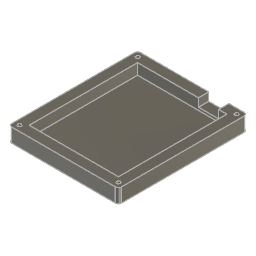
hackpad (Autodesk Fusion 360 archive; units mm, degrees)
design "case_bottom"
part number: 2026-02-01-13-29-20-341
part number: 2026-02-01-13-33-14-051
Autodesk Fusion 360 part; units mm, degrees
sketch "Sketch1" plane through (0, 0, 0) normal (0, 0, 1) x (1, 0, 0) in component "Oliver's Epic Mathpad"
  line L0 (-38.0199, 45) -> (43.9801, 45)
  line L1 (43.9801, 45) -> (43.9801, -54.6)
  line L2 (43.9801, -54.6) -> (-38.0199, -54.6)
  line L3 (-38.0199, -54.6) -> (-38.0199, 45)
  line L4 (-47.5199, 54.5) -> (53.4801, 54.5)
  line L5 (53.4801, 54.5) -> (53.4801, -64.1)
  line L6 (53.4801, -64.1) -> (-47.5199, -64.1)
  line L7 (-47.5199, -64.1) -> (-47.5199, 54.5)
  circle A0 centre (-42.5199, -59.1) radius 1.7
  circle A1 centre (48.4801, -59.1) radius 1.7
  circle A2 centre (48.4801, 49.5) radius 1.7
  circle A3 centre (-42.5199, 49.5) radius 1.7
  circle A4 centre (-42.5199, 49.5) radius 3
  circle A5 centre (48.4801, 49.5) radius 3
  circle A6 centre (48.4801, -59.1) radius 3
  circle A7 centre (-42.5199, -59.1) radius 3
  line L8 (24.7733, 2.0894) -> (-18.718, 2.1117) construction
  line L9 (-18.718, 2.1117) -> (-18.7128, 12.1117) construction
  line L10 (-18.7128, 12.1117) -> (24.7785, 12.0894) construction
  line L11 (24.7785, 12.0894) -> (24.7733, 2.0894) construction
  dimension "d1" = 82
  dimension "d2" = 99.6
  dimension "d3" = 101
  dimension "d4" = 118.6
  dimension "d5" = 9.5
  dimension "d6" = 9.5
  dimension "d7" = 3.4
  dimension "d8" = 5
  dimension "d9" = 5
  dimension "d10" = 3.4
  dimension "d11" = 5
  dimension "d12" = 5
  dimension "d13" = 3.4
  dimension "d14" = 5
  dimension "d15" = 5
  dimension "d16" = 3.4
  dimension "d17" = 5
  dimension "d18" = 5
  dimension "d19" = 6
  dimension "d20" = 6
  dimension "d21" = 6
  dimension "d22" = 6
  dimension "d39" = 3
  dimension "d41" = 10
  dimension "d42" = 28.8045
  text T0 "Oliver's Epic Mathpad" font "Arial" height 3 align left top in box 43.4913 x 10 at (24.7733, 2.0894) x (-1, 0.000513) y (0.000513, 1) spacing 1 kerned
  constraint horizontal L0
  constraint vertical L1
  constraint horizontal L2
  constraint vertical L3
  constraint horizontal L4
  constraint vertical L5
  constraint horizontal L6
  constraint vertical L7
  constraint concentric A3 A4
  constraint concentric A2 A5
  constraint concentric A1 A6
  constraint concentric A0 A7
  measures "d1" distance of L0.start L0.end
  measures "d2" distance of L0.start L2.end
  measures "d3" distance of L4.start L4.end
  measures "d4" distance of L4.start L6.end
  measures "d5" distance of L0 L4
  measures "d6" distance of L3 L7
  measures "d7" diameter of A0
  measures "d8" distance of L6 A0.centre
  measures "d9" distance of L7 A0.centre
  measures "d10" diameter of A1
  measures "d11" distance of L5 A1.centre
  measures "d12" distance of L6 A1.centre
  measures "d13" diameter of A2
  measures "d14" distance of L5 A2.centre
  measures "d15" distance of L4 A2.centre
  measures "d16" diameter of A3
  measures "d17" distance of L7 A3.centre
  measures "d18" distance of L4 A3.centre
  measures "d19" diameter of A4
  measures "d20" diameter of A5
  measures "d21" diameter of A6
  measures "d22" diameter of A7
extrude "Extrude1" add sketch "Sketch1" along normal blind 9.9 from surface at 3.1 contours A4 | A5 | A6 | A7 makes body 1 at (-45.5162, 49.3505, 9.7) makes body 2 at (-39.5236, -59.2495, 9.7) makes body 3 at (45.4838, 49.3505, 9.7) makes body 4 at (51.4764, -59.2495, 9.7) in component "Oliver's Epic Mathpad"
extrude "Extrude2" add sketch "Sketch1" along normal blind 13 contours L4 L5 L6 L7 bodies 1 2 3 4 in component "Oliver's Epic Mathpad"
extrude "Extrude3" add sketch "Sketch1" along normal blind 3 contours L0 L1 L2 L3 bodies 1 in component "Oliver's Epic Mathpad"
sketch "Sketch2" plane through (0, 0, 13) normal (0, 0, 1) x (-1, 0, 0) in component "Oliver's Epic Mathpad"
  circle A0 centre (42.5199, -49.5) radius 1.7
  circle A1 centre (-48.4801, 59.1) radius 1.7
  line L0 (-43.9801, 54.6) -> (38.0199, 54.6)
  line L1 (38.0199, 54.6) -> (38.0199, -45)
  line L2 (38.0199, -45) -> (-43.9801, -45)
  line L3 (-43.9801, -45) -> (-43.9801, 54.6)
  line L4 (47.5199, 64.1) -> (-53.4801, 64.1)
  line L5 (-53.4801, 64.1) -> (-53.4801, -54.5)
  line L6 (-53.4801, -54.5) -> (47.5199, -54.5)
  line L7 (47.5199, -54.5) -> (47.5199, 64.1)
  circle A2 centre (42.5199, 59.1) radius 1.7
  circle A3 centre (-48.4801, -49.5) radius 1.7
  line L8 (-17.9301, -54.5) -> (-36.4301, -54.5)
  line L9 (-36.4301, -54.5) -> (-36.4301, -45)
  line L10 (-36.4301, -45) -> (-17.9301, -45)
  line L11 (-17.9301, -45) -> (-17.9301, -54.5)
  line L12 (47.5199, 64.1) -> (47.5199, -54.5)
  dimension "d30" = 18.5
  dimension "d31" = 9.5
  dimension "d32" = 65.45
  constraint horizontal L8
  constraint vertical L9
  constraint horizontal L10
  constraint vertical L11
  constraint coincident L6 L8.start
  measures "d30" distance of L8.start L8.end
  measures "d31" distance of L8.start L10.end
  measures "d32" distance of L11 L12
extrude "Extrude4" cut sketch "Sketch2" against normal blind 7.5 contours L2 L6 L8 L9 L10 L11 bodies 1 in component "Oliver's Epic Mathpad"
fillet "Fillet1" radius 3 1 edges at (53.4801, -64.1, 6.5) on bodies 1 in component "Oliver's Epic Mathpad"
fillet "Fillet2" radius 3 3 edges at (-47.5199, -64.1, 6.5) (-47.5199, 54.5, 6.5) (53.4801, 54.5, 6.5) on bodies 1 in component "Oliver's Epic Mathpad"
extrude "Extrude5" add sketch "Sketch1" against normal blind 0.2 text T0 bodies 1 in component "Oliver's Epic Mathpad"
component "Oliver's Epic Mathpad" placed x (1, 0, 0) y (0, 1, 0) z (0, 0, 1) at (0, 0, 0)
equation "d32 = 59.7 mm + 5.75 mm"
equation "d40 = 'Oliver\\'s Epic Mathpad'"

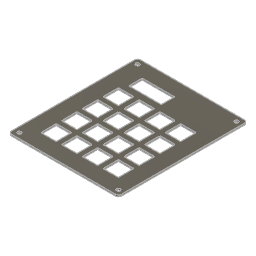
design "case_top"
part number: 2026-02-01-13-28-56-675
Autodesk Fusion 360 part; units mm, degrees
sketch "plate-2026-02-01T19_27_24.692Z" plane through (0, 0, 0) normal (0, 0, 1) x (1, 0, 0)
  line L0 (3.025, -21.575) -> (16.025, -21.575)
  line L1 (3.025, -35.575) -> (16.025, -35.575)
  line L2 (2.525, -22.075) -> (2.525, -35.075)
  line L3 (16.525, -22.075) -> (16.525, -35.075)
  arc A0 (3.025, -21.575) -> (2.525, -22.075) centre (3.025, -22.075) ccw
  arc A1 (16.525, -22.075) -> (16.025, -21.575) centre (16.025, -22.075) ccw
  arc A2 (2.525, -35.075) -> (3.025, -35.575) centre (3.025, -35.075) ccw
  arc A3 (16.025, -35.575) -> (16.525, -35.075) centre (16.025, -35.075) ccw
  line L4 (22.075, -21.575) -> (35.075, -21.575)
  line L5 (22.075, -35.575) -> (35.075, -35.575)
  line L6 (21.575, -22.075) -> (21.575, -35.075)
  line L7 (35.575, -22.075) -> (35.575, -35.075)
  arc A4 (22.075, -21.575) -> (21.575, -22.075) centre (22.075, -22.075) ccw
  arc A5 (35.575, -22.075) -> (35.075, -21.575) centre (35.075, -22.075) ccw
  arc A6 (21.575, -35.075) -> (22.075, -35.575) centre (22.075, -35.075) ccw
  arc A7 (35.075, -35.575) -> (35.575, -35.075) centre (35.075, -35.075) ccw
  line L8 (41.125, -21.575) -> (54.125, -21.575)
  line L9 (41.125, -35.575) -> (54.125, -35.575)
  line L10 (40.625, -22.075) -> (40.625, -35.075)
  line L11 (54.625, -22.075) -> (54.625, -35.075)
  arc A8 (41.125, -21.575) -> (40.625, -22.075) centre (41.125, -22.075) ccw
  arc A9 (54.625, -22.075) -> (54.125, -21.575) centre (54.125, -22.075) ccw
  arc A10 (40.625, -35.075) -> (41.125, -35.575) centre (41.125, -35.075) ccw
  arc A11 (54.125, -35.575) -> (54.625, -35.075) centre (54.125, -35.075) ccw
  line L12 (60.175, -21.575) -> (73.175, -21.575)
  line L13 (60.175, -35.575) -> (73.175, -35.575)
  line L14 (59.675, -22.075) -> (59.675, -35.075)
  line L15 (73.675, -22.075) -> (73.675, -35.075)
  arc A12 (60.175, -21.575) -> (59.675, -22.075) centre (60.175, -22.075) ccw
  arc A13 (73.675, -22.075) -> (73.175, -21.575) centre (73.175, -22.075) ccw
  arc A14 (59.675, -35.075) -> (60.175, -35.575) centre (60.175, -35.075) ccw
  arc A15 (73.175, -35.575) -> (73.675, -35.075) centre (73.175, -35.075) ccw
  line L16 (3.025, -40.625) -> (16.025, -40.625)
  line L17 (3.025, -54.625) -> (16.025, -54.625)
  line L18 (2.525, -41.125) -> (2.525, -54.125)
  line L19 (16.525, -41.125) -> (16.525, -54.125)
  arc A16 (3.025, -40.625) -> (2.525, -41.125) centre (3.025, -41.125) ccw
  arc A17 (16.525, -41.125) -> (16.025, -40.625) centre (16.025, -41.125) ccw
  arc A18 (2.525, -54.125) -> (3.025, -54.625) centre (3.025, -54.125) ccw
  arc A19 (16.025, -54.625) -> (16.525, -54.125) centre (16.025, -54.125) ccw
  line L20 (22.075, -40.625) -> (35.075, -40.625)
  line L21 (22.075, -54.625) -> (35.075, -54.625)
  line L22 (21.575, -41.125) -> (21.575, -54.125)
  line L23 (35.575, -41.125) -> (35.575, -54.125)
  arc A20 (22.075, -40.625) -> (21.575, -41.125) centre (22.075, -41.125) ccw
  arc A21 (35.575, -41.125) -> (35.075, -40.625) centre (35.075, -41.125) ccw
  arc A22 (21.575, -54.125) -> (22.075, -54.625) centre (22.075, -54.125) ccw
  arc A23 (35.075, -54.625) -> (35.575, -54.125) centre (35.075, -54.125) ccw
  line L24 (41.125, -40.625) -> (54.125, -40.625)
  line L25 (41.125, -54.625) -> (54.125, -54.625)
  line L26 (40.625, -41.125) -> (40.625, -54.125)
  line L27 (54.625, -41.125) -> (54.625, -54.125)
  arc A24 (41.125, -40.625) -> (40.625, -41.125) centre (41.125, -41.125) ccw
  arc A25 (54.625, -41.125) -> (54.125, -40.625) centre (54.125, -41.125) ccw
  arc A26 (40.625, -54.125) -> (41.125, -54.625) centre (41.125, -54.125) ccw
  arc A27 (54.125, -54.625) -> (54.625, -54.125) centre (54.125, -54.125) ccw
  line L28 (60.175, -40.625) -> (73.175, -40.625)
  line L29 (60.175, -54.625) -> (73.175, -54.625)
  line L30 (59.675, -41.125) -> (59.675, -54.125)
  line L31 (73.675, -41.125) -> (73.675, -54.125)
  arc A28 (60.175, -40.625) -> (59.675, -41.125) centre (60.175, -41.125) ccw
  arc A29 (73.675, -41.125) -> (73.175, -40.625) centre (73.175, -41.125) ccw
  arc A30 (59.675, -54.125) -> (60.175, -54.625) centre (60.175, -54.125) ccw
  arc A31 (73.175, -54.625) -> (73.675, -54.125) centre (73.175, -54.125) ccw
  line L32 (3.025, -59.675) -> (16.025, -59.675)
  line L33 (3.025, -73.675) -> (16.025, -73.675)
  line L34 (2.525, -60.175) -> (2.525, -73.175)
  line L35 (16.525, -60.175) -> (16.525, -73.175)
  arc A32 (3.025, -59.675) -> (2.525, -60.175) centre (3.025, -60.175) ccw
  arc A33 (16.525, -60.175) -> (16.025, -59.675) centre (16.025, -60.175) ccw
  arc A34 (2.525, -73.175) -> (3.025, -73.675) centre (3.025, -73.175) ccw
  arc A35 (16.025, -73.675) -> (16.525, -73.175) centre (16.025, -73.175) ccw
  line L36 (22.075, -59.675) -> (35.075, -59.675)
  line L37 (22.075, -73.675) -> (35.075, -73.675)
  line L38 (21.575, -60.175) -> (21.575, -73.175)
  line L39 (35.575, -60.175) -> (35.575, -73.175)
  arc A36 (22.075, -59.675) -> (21.575, -60.175) centre (22.075, -60.175) ccw
  arc A37 (35.575, -60.175) -> (35.075, -59.675) centre (35.075, -60.175) ccw
  arc A38 (21.575, -73.175) -> (22.075, -73.675) centre (22.075, -73.175) ccw
  arc A39 (35.075, -73.675) -> (35.575, -73.175) centre (35.075, -73.175) ccw
  line L40 (41.125, -59.675) -> (54.125, -59.675)
  line L41 (41.125, -73.675) -> (54.125, -73.675)
  line L42 (40.625, -60.175) -> (40.625, -73.175)
  line L43 (54.625, -60.175) -> (54.625, -73.175)
  arc A40 (41.125, -59.675) -> (40.625, -60.175) centre (41.125, -60.175) ccw
  arc A41 (54.625, -60.175) -> (54.125, -59.675) centre (54.125, -60.175) ccw
  arc A42 (40.625, -73.175) -> (41.125, -73.675) centre (41.125, -73.175) ccw
  arc A43 (54.125, -73.675) -> (54.625, -73.175) centre (54.125, -73.175) ccw
  line L44 (60.175, -59.675) -> (73.175, -59.675)
  line L45 (60.175, -73.675) -> (73.175, -73.675)
  line L46 (59.675, -60.175) -> (59.675, -73.175)
  line L47 (73.675, -60.175) -> (73.675, -73.175)
  arc A44 (60.175, -59.675) -> (59.675, -60.175) centre (60.175, -60.175) ccw
  arc A45 (73.675, -60.175) -> (73.175, -59.675) centre (73.175, -60.175) ccw
  arc A46 (59.675, -73.175) -> (60.175, -73.675) centre (60.175, -73.175) ccw
  arc A47 (73.175, -73.675) -> (73.675, -73.175) centre (73.175, -73.175) ccw
  line L48 (3.025, -78.725) -> (16.025, -78.725)
  line L49 (3.025, -92.725) -> (16.025, -92.725)
  line L50 (2.525, -79.225) -> (2.525, -92.225)
  line L51 (16.525, -79.225) -> (16.525, -92.225)
  arc A48 (3.025, -78.725) -> (2.525, -79.225) centre (3.025, -79.225) ccw
  arc A49 (16.525, -79.225) -> (16.025, -78.725) centre (16.025, -79.225) ccw
  arc A50 (2.525, -92.225) -> (3.025, -92.725) centre (3.025, -92.225) ccw
  arc A51 (16.025, -92.725) -> (16.525, -92.225) centre (16.025, -92.225) ccw
  line L52 (22.075, -78.725) -> (35.075, -78.725)
  line L53 (22.075, -92.725) -> (35.075, -92.725)
  line L54 (21.575, -79.225) -> (21.575, -92.225)
  line L55 (35.575, -79.225) -> (35.575, -92.225)
  arc A52 (22.075, -78.725) -> (21.575, -79.225) centre (22.075, -79.225) ccw
  arc A53 (35.575, -79.225) -> (35.075, -78.725) centre (35.075, -79.225) ccw
  arc A54 (21.575, -92.225) -> (22.075, -92.725) centre (22.075, -92.225) ccw
  arc A55 (35.075, -92.725) -> (35.575, -92.225) centre (35.075, -92.225) ccw
  line L56 (41.125, -78.725) -> (54.125, -78.725)
  line L57 (41.125, -92.725) -> (54.125, -92.725)
  line L58 (40.625, -79.225) -> (40.625, -92.225)
  line L59 (54.625, -79.225) -> (54.625, -92.225)
  arc A56 (41.125, -78.725) -> (40.625, -79.225) centre (41.125, -79.225) ccw
  arc A57 (54.625, -79.225) -> (54.125, -78.725) centre (54.125, -79.225) ccw
  arc A58 (40.625, -92.225) -> (41.125, -92.725) centre (41.125, -92.225) ccw
  arc A59 (54.125, -92.725) -> (54.625, -92.225) centre (54.125, -92.225) ccw
  line L60 (60.175, -78.725) -> (73.175, -78.725)
  line L61 (60.175, -92.725) -> (73.175, -92.725)
  line L62 (59.675, -79.225) -> (59.675, -92.225)
  line L63 (73.675, -79.225) -> (73.675, -92.225)
  arc A60 (60.175, -78.725) -> (59.675, -79.225) centre (60.175, -79.225) ccw
  arc A61 (73.675, -79.225) -> (73.175, -78.725) centre (73.175, -79.225) ccw
  arc A62 (59.675, -92.225) -> (60.175, -92.725) centre (60.175, -92.225) ccw
  arc A63 (73.175, -92.725) -> (73.675, -92.225) centre (73.175, -92.225) ccw
  line L64 (-12.4, 10.954) -> (88.6, 10.954)
  line L65 (88.6, 10.954) -> (88.6, -107.646)
  line L66 (88.6, -107.646) -> (-12.4, -107.646)
  line L67 (-12.4, -107.646) -> (-12.4, 10.954)
  line L68 (5.796, -3.011) -> (35.396, -3.011)
  line L69 (35.396, -3.011) -> (35.396, -15.111)
  line L70 (35.396, -15.111) -> (5.796, -15.111)
  line L71 (5.796, -15.111) -> (5.796, -3.011)
  circle A64 centre (83.6, 5.954) radius 1.7
  circle A65 centre (-7.4, 5.954) radius 1.7
  circle A66 centre (-7.4, -102.646) radius 1.7
  circle A67 centre (83.6, -102.646) radius 1.7
  dimension "d3" = 101
  dimension "d4" = 118.6
  dimension "d6" = 14.925
  dimension "d7" = 14.921
  dimension "d8" = 29.6
  dimension "d9" = 12.1
  dimension "d10" = 13.965
  dimension "d11" = 18.196
  dimension "d12" = 3.4
  dimension "d13" = 5
  dimension "d14" = 5
  dimension "d15" = 3.4
  dimension "d16" = 5
  dimension "d17" = 5
  dimension "d18" = 3.4
  dimension "d19" = 5
  dimension "d20" = 5
  dimension "d21" = 3.4
  dimension "d22" = 5
  dimension "d23" = 5
  constraint horizontal L64
  constraint vertical L65
  constraint horizontal L66
  constraint vertical L67
  constraint horizontal L68
  constraint vertical L69
  constraint horizontal L70
  constraint vertical L71
  measures "d3" distance of L64.start L64.end
  measures "d4" distance of L64.start L66.end
  measures "d6" distance of L18 L67
  measures "d7" distance of L49 L66
  measures "d8" distance of L68.start L68.end
  measures "d9" distance of L68.start L70.end
  measures "d10" distance of L64 L68
  measures "d11" distance of L67 L71
  measures "d12" diameter of A64
  measures "d13" distance of L64 A64.centre
  measures "d14" distance of L65 A64.centre
  measures "d15" diameter of A65
  measures "d16" distance of L64 A65.centre
  measures "d17" distance of L67 A65.centre
  measures "d18" diameter of A66
  measures "d19" distance of L66 A66.centre
  measures "d20" distance of L67 A66.centre
  measures "d21" diameter of A67
  measures "d22" distance of L65 A67.centre
  measures "d23" distance of L66 A67.centre
extrude "Extrude1" add sketch "plate-2026-02-01T19_27_24.692Z" along normal blind 1.5
fillet "Fillet1" radius 3 4 edges at (88.6, -107.646, 0.75) (88.6, 10.954, 0.75) (-12.4, 10.954, 0.75) (-12.4, -107.646, 0.75)
equation "d6 = 4.925 mm + 10 mm"
equation "d7 = 4.921 mm + 10 mm"
equation "d10 = 10 mm + 4.015 mm - 0.05 mm"
equation "d11 = 10 mm + 8.246 mm - 0.05 mm"
